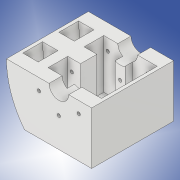
# Autodesk Inventor part: SJ005
Saved by Autodesk Inventor 2017 SP1 (Build 210196100, 196)
## iProperties
Created: 2017-06-04
Part Number: SJ005
Material: ABS Plastic
Document SubType Name: Modeling
Designer: Zach
Density: 1.06 g/cm^3
Appearance: CR White
Author: Zach
Autodesk Inventor part; units mm, degrees
ref_plane "YZ Plane" through (0, 0, 0) normal (1, 0, 0) x (0, 1, 0)
ref_plane "XZ Plane" through (0, 0, 0) normal (0, 1, 0) x (-1, 0, 0)
ref_plane "XY Plane" through (0, 0, 0) normal (0, 0, 1) x (1, 0, 0)
sketch "Sketch1" plane through (0, 0, 0) normal (0, 0, 1) x (1, 0, 0)
  circle A0 centre (0, 80) radius 130 construction
  line L0 (0, -50) -> (0, 0) construction
  line L1 (0, 0) -> (-102.4695, 0) construction
  arc A1 (-130, 80) -> (-102.4695, 0) centre (0, 80) ccw
  line L2 (-130, 80) -> (0, 80)
  line L3 (0, 80) -> (0, 0)
  line L4 (-102.4695, 0) -> (0, 0)
  dimension "d0" = 260
  dimension "d1" = 50
  constraints: 10 end point, 5 point on circle, 2 centre point, 2 perpendicular, 1 coincident, 1 collinear, 1 concentric, 1 horizontal, 1 vertical
  measures "d0" diameter of A0
  measures "d1" distance of L0.start L0.end
extrude "Extrusion1" add sketch "Sketch1" along normal blind 125
sketch "Sketch6" plane through (-130, 80, 0) normal (0, 1, 0) x (1, 0, 0)
  line L0 (0, 0) -> (0, -125) projected
  line L1 (0, 0) -> (130, 0)
  line L2 (130, 0) -> (130, -125)
  line L3 (130, -125) -> (0, -125)
  line L4 (0, -125) -> (0, 0)
  line L5 (5, -120) -> (125, -120)
  line L6 (125, -120) -> (125, -5)
  line L7 (125, -5) -> (5, -5)
  line L8 (5, -5) -> (5, -120)
  point P0 (130, 0)
  dimension "d25" = 5
  constraints: 16 end point, 4 parallel, 2 perpendicular, 1 horizontal, 3 other
  measures "d25" distance between parallel lines of L3 L5
extrude "Extrusion5" cut sketch "Sketch6" against normal blind 75 contours L8 L7 L6 L5
sketch "Sketch7" plane through (-102.4695, 0, 0) normal (0, -1, 0) x (1, 0, 0)
  circle A0 centre (35, 97.53) radius 2.5
  circle A1 centre (85, 97.53) radius 2.5
  line L0 (0, 125) -> (102.4695, 125) projected
  line L1 (0, 0) -> (0, 125) projected
  circle A2 centre (35, 27.53) radius 2.5
  circle A3 centre (85, 27.53) radius 2.5
  line L2 (102.4695, 0) -> (102.4695, 125) projected
  dimension "d28" = 5
  dimension "d29" = 5
  dimension "d30" = 27.47
  dimension "d31" = 50
  dimension "d33" = 5
  dimension "d34" = 5
  dimension "d35" = 70
  dimension "d82" = 35
  constraints: 4 centre point, 2 horizontal alignment, 2 vertical alignment
  measures "d28" diameter of A0
  measures "d29" diameter of A1
  measures "d30" distance from line of L0 A0.centre
  measures "d31" distance of A1.centre A0.centre
  measures "d33" diameter of A2
  measures "d34" diameter of A3
  measures "d35" distance of A2.centre A0.centre
  measures "d82" horizontal distance of L0.start A0.centre
extrude "Extrusion6" cut sketch "Sketch7" against normal through all
sketch "Sketch8" plane through (0, 0, 125) normal (0, 0, 1) x (1, 0, 0)
  line L0 (0, 80) -> (-130, 80) projected
  arc A0 (-130, 80) -> (-102.4695, 0) centre (0, 80) ccw projected
  arc A1 (-130, 80) -> (-102.4695, 0) centre (9.9581, 83.4269) ccw
  line L1 (-102.4695, 0) -> (-97.4695, 0)
  line L2 (-102.4695, 0) -> (0, 0) projected
  line L3 (-130, 80) -> (-125, 80)
  arc A2 (-125, 80) -> (-97.4695, 0) centre (14.9581, 83.4269) ccw
  dimension "d40" = 5
  dimension "d41" = 5
  dimension "d42" = 140
  constraints: 4 end point, 4 point on circle, 2 centre point, 2 point on line
  measures "d40" distance of L1.start L1.end
  measures "d41" distance of L0.end L3.end
  measures "d42" radius of A2
extrude "Extrusion7" add sketch "Sketch8" against normal blind 125
sketch "Sketch11" plane through (-130, 5, 0) normal (0, 1, 0) x (1, 0, 0)
  line L0 (125, -5) -> (125, -120) projected
  line L1 (125, -50) -> (5, -50)
  line L2 (5, -50) -> (5, -65)
  line L3 (5, -65) -> (125, -65)
  line L4 (125, -65) -> (125, -50)
  line L5 (125, -60) -> (5, -60)
  line L6 (5, -60) -> (5, -75)
  line L7 (5, -75) -> (125, -75)
  line L8 (125, -75) -> (125, -60)
  line L9 (32.7619, 0) -> (32.7619, -150)
  line L10 (125, -105) -> (5, -105)
  line L11 (5, -105) -> (5, -120)
  line L12 (5, -120) -> (125, -120)
  line L13 (125, -120) -> (125, -105)
  line L14 (125, -20) -> (5, -20)
  line L15 (5, -20) -> (5, -5)
  line L16 (5, -5) -> (125, -5)
  line L17 (125, -5) -> (125, -20)
  line L18 (5, -5) -> (125, -5)
  line L19 (5, -120) -> (5, -5) projected
  line L20 (125, -120) -> (5, -120) projected
  line L21 (125, -5) -> (125, -20)
  point P0 (130, 0)
  point P1 (65, -120)
  point P2 (65, -5)
  point P3 (5, -12.5)
  point P4 (5, -57.5)
  dimension "d54" = 15
  dimension "d55" = 15
  dimension "d56" = 15
  dimension "d57" = 15
  dimension "d58" = 30
  dimension "d59" = 30
  dimension "d66" = 5
  constraints: 38 end point, 8 parallel, 8 point on line, 6 midpoint, 4 horizontal, 4 perpendicular, 1 collinear
  measures "d54" distance of L2.end L1.end
  measures "d55" distance of L6.end L5.end
  measures "d56" distance between parallel lines of L12 L10
  measures "d57" distance between parallel lines of L16 L14
  measures "d58" distance between parallel lines of L14 L1
  measures "d59" distance between parallel lines of L10 L7
  measures "d66" distance from line of point (130, 0) L18
extrude "Extrusion10" add sketch "Sketch11" along normal blind 75 contours L0 L14 L9 L16 | L9 L14 L15 L16 | L0 L5 L9 L1 | L0 L3 L9 L5 | L9 L5 L2 L1 | L0 L7 L9 L3 | L9 L3 L2 L5 | L9 L7 L6 L3 | L0 L12 L9 L10 | L9 L12 L11 L10
sketch "Sketch12" plane through (-130, 5, 0) normal (0, 1, 0) x (1, 0, 0)
  line L0 (27.5305, 0) -> (130, 0) projected
  line L1 (27.5305, -125) -> (130, -125) projected
  line L2 (72.5, 0) -> (87.5, 0)
  line L3 (87.5, 0) -> (87.5, -125)
  line L4 (87.5, -125) -> (72.5, -125)
  line L5 (72.5, -125) -> (72.5, 0)
  line L6 (28.5256, 0) -> (43.5256, 0)
  line L7 (43.5256, 0) -> (43.5256, -125)
  line L8 (43.5256, -125) -> (28.5256, -125)
  line L9 (28.5256, -125) -> (28.5256, 0)
  line L10 (130, 0) -> (130, -125) projected
  dimension "d62" = 15
  dimension "d63" = 15
  dimension "d92" = 42.5
  constraints: 16 end point, 4 parallel, 4 point on line, 2 horizontal, 2 perpendicular
  measures "d62" distance of L3.end L4.end
  measures "d63" distance of L7.end L8.end
  measures "d92" distance between parallel lines of L10 L3
extrude "Extrusion11" add sketch "Sketch12" along normal blind 75 contours L0 L7 L1 L9 | L0 L3 L1 L5
sketch "Sketch9" plane through (0, 0, 125) normal (0, 0, 1) x (1, 0, 0)
  circle A0 centre (-50, 80) radius 15
  point P0 (0, 0)
  point P1 (0, 80)
  dimension "d45" = 30
  dimension "d46" = 50
  constraints: 1 centre point, 1 horizontal alignment
  measures "d45" diameter of A0
  measures "d46" horizontal distance of A0.centre point (0, 0)
extrude "Extrusion8" cut sketch "Sketch9" against normal through all
sketch "Sketch13" plane through (0, 0, 0) normal (0, 0, -1) x (-1, 0, 0)
  arc A0 (102.4695, 0) -> (130, 80) centre (-9.9581, 83.4269) ccw
  line L0 (130, 80) -> (130, 80)
  arc A1 (102.4695, 0) -> (130, 80) centre (0, 80) ccw projected
  line L1 (130, 80) -> (130, 80)
  line L2 (65, 80) -> (130, 80) projected
  line L3 (130, 80) -> (130, 0)
  line L4 (130, 0) -> (102.4695, 0)
  point P0 (0, 0)
  dimension "d67" = 140
  constraints: 8 end point, 2 perpendicular, 2 point on circle, 2 vertical, 1 centre point, 1 tangent
  measures "d67" radius of A0
extrude "Extrusion12" cut sketch "Sketch13" against normal through all contours A1 L3 L4
sketch "Sketch14" plane through (0, 0, 125) normal (0, 0, 1) x (1, 0, 0)
  line L0 (-102.4695, 0) -> (0, 0) construction
  line L1 (-50, 0) -> (-50, 196.0469) construction
  line L2 (0, 80) -> (-93.0222, 80) construction
  line L3 (-50, 80) -> (28.9192, 80) construction
  circle A0 centre (-50, 115) radius 2.5
  circle A1 centre (-50, 80) radius 35 construction
  circle A2 centre (-80.3109, 97.5) radius 2.5
  circle A3 centre (-80.3109, 62.5) radius 2.5
  circle A4 centre (-50, 45) radius 2.5
  circle A5 centre (-19.6891, 62.5) radius 2.5
  circle A6 centre (-19.6891, 97.5) radius 2.5
  dimension "d74" = 70
  dimension "d70" = 50
  dimension "d72" = 5
  dimension "d77" = 360
  constraints: 6 centre point, 6 end point, 4 point on line, 2 horizontal, 1 coincident, 1 perpendicular, 1 vertical alignment, 15 other
  measures "d70" distance from line of L0.end L1
  measures "d72" diameter of A0
extrude "Extrusion13" cut sketch "Sketch14" against normal through all contours A3 | A4 | A5
sketch "Sketch16" plane through (-102.4695, 0, 0) normal (0, -1, 0) x (1, 0, 0)
  line L0 (35.4695, 31.5) -> (35.4695, 93.5) construction
  line L1 (97.4695, 93.5) -> (35.4695, 93.5) construction
  line L2 (35.4695, 93.5) -> (35.4695, 31.5) construction
  line L3 (35.4695, 31.5) -> (97.4695, 31.5) construction
  line L4 (97.4695, 31.5) -> (97.4695, 93.5) construction
  line L5 (0, 125) -> (102.4695, 125) projected
  line L6 (0, 0) -> (102.4695, 0) projected
  line L7 (102.4695, 0) -> (102.4695, 125) projected
  line L8 (97.4695, 93.5) -> (92.4695, 93.5) construction
  line L9 (92.4695, 93.5) -> (92.4695, 88.5) construction
  line L10 (92.4695, 88.5) -> (97.4695, 88.5) construction
  line L11 (97.4695, 88.5) -> (97.4695, 93.5) construction
  line L12 (35.4695, 31.5) -> (40.4695, 31.5) construction
  line L13 (40.4695, 31.5) -> (40.4695, 36.5) construction
  line L14 (40.4695, 36.5) -> (35.4695, 36.5) construction
  line L15 (35.4695, 36.5) -> (35.4695, 31.5) construction
  line L16 (35.4695, 93.5) -> (40.4695, 93.5) construction
  line L17 (40.4695, 93.5) -> (40.4695, 88.5) construction
  line L18 (40.4695, 88.5) -> (35.4695, 88.5) construction
  line L19 (35.4695, 88.5) -> (35.4695, 93.5) construction
  line L20 (97.4695, 31.5) -> (92.4695, 31.5) construction
  line L21 (92.4695, 31.5) -> (92.4695, 36.5) construction
  line L22 (92.4695, 36.5) -> (97.4695, 36.5) construction
  line L23 (97.4695, 36.5) -> (97.4695, 31.5) construction
  line L24 (92.4695, 93.5) -> (40.4695, 93.5)
  line L25 (40.4695, 88.5) -> (40.4695, 93.5)
  line L26 (35.4695, 88.5) -> (40.4695, 88.5)
  line L27 (35.4695, 88.5) -> (35.4695, 36.5)
  line L28 (35.4695, 36.5) -> (40.4695, 36.5)
  line L29 (40.4695, 36.5) -> (40.4695, 31.5)
  line L30 (40.4695, 31.5) -> (92.4695, 31.5)
  line L31 (92.4695, 31.5) -> (92.4695, 36.5)
  line L32 (92.4695, 36.5) -> (97.4695, 36.5)
  line L33 (97.4695, 20) -> (97.4695, 50) projected
  line L34 (97.4695, 36.5) -> (97.4695, 88.5)
  line L35 (97.4695, 75) -> (97.4695, 105) projected
  line L36 (92.4695, 88.5) -> (97.4695, 88.5)
  line L37 (92.4695, 88.5) -> (92.4695, 93.5)
  point P0 (97.4695, 62.5)
  point P1 (102.4695, 62.5)
  point P2 (66.4695, 31.5)
  point P3 (51.2348, 0)
  dimension "d100" = 62
  dimension "d101" = 62
  dimension "d102" = 5
  dimension "d103" = 5
  dimension "d104" = 5
  dimension "d105" = 5
  dimension "d106" = 5
  dimension "d107" = 5
  dimension "d108" = 5
  dimension "d109" = 5
  dimension "d110" = 5
  constraints: 66 end point, 13 perpendicular, 9 parallel, 6 horizontal, 4 midpoint, 3 collinear, 1 horizontal alignment, 1 vertical
  measures "d100" distance of L0.start L0.end
  measures "d101" distance of L0.start L3.end
  measures "d102" distance between parallel lines of L7 L4
  measures "d103" distance of L10.end L9.end
  measures "d104" distance of L9.end L8.end
  measures "d105" distance of L14.end L13.end
  measures "d106" distance of L13.end L12.end
  measures "d107" distance of L17.end L18.end
  measures "d108" distance of L16.end L17.end
  measures "d109" distance of L21.end L22.end
  measures "d110" distance of L20.end L21.end
extrude "Extrusion15" cut sketch "Sketch16" against normal through all
equation "\"d101\" = d100"
body "Solid1"
